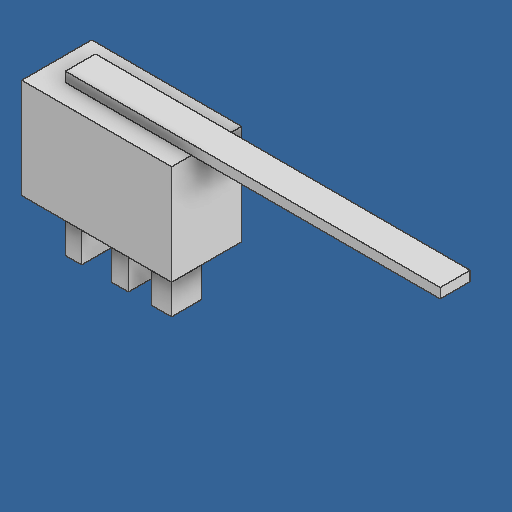
# Autodesk Inventor part: limit_switch
Saved by Autodesk Inventor 2026.2 (Build 302298000, 298)
## iProperties
Created: 2026-01-30
Part Number: limit_switch
Material: Generic
Document SubType Name: Modeling
Designer: Thoma
Density: 1 g/cm^3
Appearance: Default
Author: Thoma
Autodesk Inventor part; units mm, degrees
ref_plane "YZ Plane" through (0, 0, 0) normal (1, 0, 0) x (0, 1, 0)
ref_plane "XZ Plane" through (0, 0, 0) normal (0, 1, 0) x (-1, 0, 0)
ref_plane "XY Plane" through (0, 0, 0) normal (0, 0, 1) x (1, 0, 0)
sketch "Sketch1" plane through (0, 0, 0) normal (0, 1, 0) x (-1, 0, 0)
  line L0 (0, 0) -> (15, 0)
  line L1 (15, 0) -> (15, -7)
  line L2 (15, -7) -> (0, -7)
  line L3 (0, -7) -> (0, 0)
  dimension "d0" = 15
  dimension "d1" = 7
  constraints: 8 end point, 2 parallel, 1 horizontal, 1 perpendicular
  measures "d0" distance of L1.end L2.end
  measures "d1" distance of L0.end L1.end
extrude "Extrusion1" add sketch "Sketch1" along normal blind 10
sketch "Sketch2" plane through (0, 10, 0) normal (0, 1, 0) x (1, 0, 0)
  line L0 (-12.6158, 4.9907) -> (24.8842, 4.9907)
  line L1 (24.8842, 4.9907) -> (24.8842, 1.9907)
  line L2 (24.8842, 1.9907) -> (-12.6158, 1.9907)
  line L3 (-12.6158, 1.9907) -> (-12.6158, 4.9907)
  point P0 (0, 0)
  dimension "d4" = 37.5
  dimension "d5" = 3
  constraints: 8 end point, 2 parallel, 1 horizontal, 1 perpendicular
  measures "d4" distance of L1.end L2.end
  measures "d5" distance of L0.end L1.end
extrude "Extrusion2" add sketch "Sketch2" along normal blind 0.98
sketch "Sketch3" plane through (0, 0, 0) normal (0, -1, 0) x (1, 0, 0)
  line L0 (-12.6158, -4.9907) -> (-12.6158, -1.9907) projected
  line L1 (0, -1.9907) -> (-12.6158, -1.9907) projected
  line L2 (-12.6158, -4.9907) -> (-11, -4.9907)
  line L3 (-11, -4.9907) -> (-11, -1.9907)
  line L4 (-11, -1.9907) -> (-12.6158, -1.9907)
  line L5 (-12.6158, -1.9907) -> (-12.6158, -4.9907)
  line L6 (-8, -4.9907) -> (-6.3079, -4.9907)
  line L7 (-6.3079, -4.9907) -> (-6.3079, -1.9907)
  line L8 (-6.3079, -1.9907) -> (-8, -1.9907)
  line L9 (-8, -1.9907) -> (-8, -4.9907)
  line L10 (-4, -4.9907) -> (-2, -4.9907)
  line L11 (-2, -4.9907) -> (-2, -1.9907)
  line L12 (-2, -1.9907) -> (-4, -1.9907)
  line L13 (-4, -1.9907) -> (-4, -4.9907)
  point P0 (0, 0)
  constraints: 24 end point, 6 parallel, 4 point on line, 3 horizontal, 3 perpendicular, 1 midpoint
extrude "Extrusion3" add sketch "Sketch3" along normal blind 5
body "Solid1"
